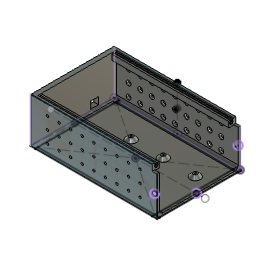
3U_Sliding_Nut (Autodesk Fusion 360 design; units mm, degrees)
Autodesk Fusion 360 part; units mm, degrees
note: some values were not read from the file. Set by a fixed rule: which face or edge a step refers to.
sketch "Sketch1" plane through (0, 0, 0) normal (0, 0, 1) x (1, 0, 0) in component "Case_Body"
  line L0 (96.52, 65) -> (-96.52, 65)
  line L1 (-96.52, 65) -> (-96.52, -65)
  line L2 (-96.52, -65) -> (96.52, -65)
  line L3 (96.52, -65) -> (96.52, 65)
  line L4 (96.52, 65) -> (-96.52, -65) construction
  line L5 (-96.52, 65) -> (96.52, -65) construction
  line L6 (-104.52, 69) -> (-96.52, 69)
  line L7 (-96.52, 69) -> (-96.52, -69)
  line L8 (-96.52, -69) -> (-104.52, -69)
  line L9 (-104.52, -69) -> (-104.52, 69)
  line L10 (-104.52, 69) -> (-96.52, -69) construction
  line L11 (-96.52, 69) -> (-104.52, -69) construction
  line L12 (-140, 0) -> (115, 0) construction
  line L13 (96.52, -69) -> (-96.52, -69)
  line L14 (-96.52, -69) -> (-96.52, -65)
  line L15 (-96.52, -65) -> (96.52, -65)
  line L16 (96.52, -65) -> (96.52, -69)
  line L17 (-96.52, 65) -> (96.52, 65)
  line L18 (-96.52, 69) -> (-96.52, 65)
  line L19 (96.52, 65) -> (96.52, 69)
  line L20 (-96.52, 65) -> (96.52, 65)
  line L21 (96.52, 69) -> (-96.52, 69)
  line L22 (104.52, 65) -> (96.52, 65)
  line L23 (96.52, 65) -> (96.52, -65)
  line L24 (96.52, -65) -> (104.52, -65)
  line L25 (104.52, -65) -> (104.52, 65)
  line L26 (104.52, 65) -> (96.52, -65) construction
  line L27 (96.52, 65) -> (104.52, -65) construction
  line L28 (104.52, 69) -> (96.52, 69)
  line L29 (96.52, 69) -> (96.52, 65)
  line L30 (96.52, 65) -> (104.52, 65)
  line L31 (104.52, 65) -> (104.52, 69)
  line L32 (96.52, -65) -> (104.52, -65)
  line L33 (104.52, -65) -> (104.52, -69)
  line L34 (104.52, -69) -> (96.52, -69)
  line L35 (96.52, -69) -> (96.52, -65)
  point P0 (-100.52, 0)
  point P1 (100.52, 0)
  dimension "d8" = 130
  dimension "d9" = 193.04
  dimension "d10" = 138
  dimension "d11" = 8
  dimension "d12" = 4
  dimension "d14" = 8
  dimension "d15" = 130
  constraint horizontal L0
  constraint perpendicular L0 L1
  constraint parallel L0 L2
  constraint parallel L1 L3
  constraint coincident L4 origin
  constraint coincident L5 origin
  constraint horizontal L6
  constraint perpendicular L6 L7
  constraint parallel L6 L8
  constraint parallel L7 L9
  constraint coincident L10 P0
  constraint coincident L11 P0
  constraint perpendicular L7 L12
  constraint coincident origin L12
  constraint coincident P0 L12
  constraint collinear L1 L7
  constraint horizontal L13
  constraint vertical L14
  constraint horizontal L15
  constraint vertical L16
  constraint coincident L1.end L2.start
  constraint symmetric L1.end L12 L0.end
  constraint symmetric L2.end L12 L0.start
  constraint symmetric L12 L13.start L19.end
  constraint symmetric L12 L7.end L6.end
  constraint symmetric L12 L1.end L0.end
  constraint symmetric L12 L2.end L0.start
  constraint horizontal L22
  constraint perpendicular L22 L23
  constraint parallel L22 L24
  constraint parallel L23 L25
  constraint coincident L26 P1
  constraint coincident L27 P1
  constraint coincident L12 P1
  constraint collinear L3 L23
  constraint horizontal L28
  constraint vertical L29
  constraint horizontal L30
  constraint vertical L31
  constraint coincident L0.start L3.end
  constraint coincident L22.start L25.end
  constraint coincident L19.end L21.start
  constraint horizontal L32
  constraint vertical L33
  constraint horizontal L34
  constraint vertical L35
  constraint coincident L2.end L3.start
  constraint coincident L13.start L16.end
  constraint coincident L24.end L25.start
  measures "d8" distance of L0.start L2.end
  measures "d9" distance of L0.start L0.end
  measures "d10" distance of L6.start L8.end
  measures "d11" distance of L7.end L8.end
  measures "d12" distance of L13.start L2.end
  measures "d14" distance of L22.start L0.start
  measures "d15" distance of L22.start L24.end
extrude "Extrude1" add sketch "Sketch1" along normal blind 4 contours L0 L1 L2 L3 L7 L15 L17 L20 L23 makes body 1 in component "Case_Body"
extrude "Extrude2" add sketch "Sketch1" along normal blind 74 contours L0 L7 L17 L18 L19 L20 L21 L29 | L1 L6 L7 L8 L9 L14 L18 | L2 L7 L13 L14 L15 L16 L35 bodies 1 in component "Case_Body"
extrude "Extrude3" add sketch "Sketch1" along normal blind 4 contours L3 L22 L23 L24 L25 L30 L32 bodies 1 in component "Case_Body"
extrude "Extrude4" add sketch "Sketch1" along normal blind 64 contours L19 L22 L28 L29 L30 L31 | L16 L24 L32 L33 L34 L35 bodies 1 in component "Case_Body"
ref_plane "WorkPlane1" through (104.52, 0, 32) normal (1, 0, 0) x (0, 1, 0) in component "Lid"
sketch "Sketch4" plane through (104.52, 0, 22) normal (1, 0, 0) x (0, 1, 0) in component "Lid"
  line L0 (-69, 42) -> (-65, 42)
  line L1 (-65, 42) -> (-65, 52)
  line L2 (-65, 52) -> (-69, 52)
  line L3 (-69, 52) -> (-69, 42)
  line L4 (65, 42) -> (69, 42)
  line L5 (69, 42) -> (69, 52)
  line L6 (69, 52) -> (65, 52)
  line L7 (65, 52) -> (65, 42)
  line L8 (-65, -18) -> (65, -18)
  line L9 (65, -18) -> (65, 52)
  line L10 (65, 52) -> (-65, 52)
  line L11 (-65, 52) -> (-65, -18)
extrude "Extrude1'" add sketch "Sketch4" against normal blind 8 separate body makes body 2 in component "Lid"
move_face "OffsetFaces1" offset -0.1 5 faces at (101.8533, -65, 44) (101.8533, -67.6667, 64) (99.1867, -21.6667, 4) (101.8533, 65, 24) (101.8533, 66.3333, 64) on bodies 2 in component "Lid"
sketch "Sketch5" plane through (0, 0, 4.1) normal (0, 0, -1) x (1, 0, 0) in component "Lid"
  line L0 (104.52, -64.9) -> (104.52, 64.9)
  line L1 (104.52, 64.9) -> (96.52, 64.9)
  line L2 (96.52, 64.9) -> (96.52, -64.9)
  line L3 (96.52, -64.9) -> (104.52, -64.9)
  line L4 (0, 0) -> (118, 0) construction
  circle A0 centre (100.52, 0) radius 1.25
  line L5 (100.52, 64.9) -> (100.52, -64.9) construction
  dimension "d29" = 2.5
  constraint coincident L4.start origin
  constraint perpendicular L2 L4
  constraint coincident L4 A0.centre
  constraint midpoint L1 L5.start
  constraint midpoint L3 L5.end
  constraint midpoint A0.centre L5
  measures "d29" diameter of A0
extrude "Extrude2'" cut sketch "Sketch5" against normal blind 10 contours A0 bodies 2 in component "Lid"
sketch "Sketch6" plane through (96.52, 0, 0) normal (-1, 0, 0) x (0, -1, 0) in component "Lid"
  line L0 (64.9, 64.1) -> (69, 64.1)
  line L1 (69, 64.1) -> (69, 74)
  line L2 (69, 74) -> (-69, 74)
  line L3 (-69, 74) -> (-69, 64.1)
  line L4 (-69, 64.1) -> (-64.9, 64.1)
  line L5 (-64.9, 64.1) -> (-64.9, 4.1)
  line L6 (-64.9, 4.1) -> (64.9, 4.1)
  line L7 (64.9, 4.1) -> (64.9, 64.1)
  line L8 (0, 0) -> (0, 41.8429) construction
  line L9 (2.55, 7.1) -> (-2.55, 7.1)
  line L10 (-2.55, 7.1) -> (-2.55, 5.5)
  line L11 (-2.55, 5.5) -> (2.55, 5.5)
  line L12 (2.55, 5.5) -> (2.55, 7.1)
  line L13 (2.55, 7.1) -> (-2.55, 5.5) construction
  line L14 (-2.55, 7.1) -> (2.55, 5.5) construction
  point P0 (0, 6.3)
  dimension "d33" = 1.6
  dimension "d34" = 3
  dimension "d35" = 5.1
  constraint coincident L8.start origin
  constraint perpendicular L6 L8
  constraint horizontal L9
  constraint perpendicular L9 L10
  constraint parallel L9 L11
  constraint parallel L10 L12
  constraint coincident L13 P0
  constraint coincident L14 P0
  constraint coincident L8 P0
  measures "d33" distance of L9.start L11.end
  measures "d34" distance of L6 L9
  measures "d35" distance of L9.start L9.end
extrude "Extrude3'" cut sketch "Sketch6" against normal blind 6.5 contours L9 L10 L11 L12 bodies 2 in component "Lid"
sketch "Sketch7" plane through (0, -64.9, 0) normal (0, -1, 0) x (1, 0, 0) in component "Lid"
  line L0 (104.52, 4.1) -> (104.52, 64.1)
  line L1 (104.52, 64.1) -> (96.52, 64.1)
  line L2 (96.52, 64.1) -> (96.52, 4.1)
  line L3 (96.52, 4.1) -> (104.52, 4.1)
  line L4 (96.52, 64.1) -> (104.52, 4.1) construction
  line L5 (104.52, 64.1) -> (96.52, 4.1) construction
  circle A0 centre (100.52, 34.1) radius 1.25
  dimension "d38" = 2.5
  constraint coincident L1.end L2.start
  constraint coincident L0.start L3.end
  constraint coincident L0.end L1.start
  constraint coincident L2.end L3.start
  constraint midpoint L4 A0.centre
  measures "d38" diameter of A0
extrude "Extrude4'" cut sketch "Sketch7" against normal blind 10 contours A0 bodies 2 in component "Lid"
sketch "Sketch8" plane through (96.52, 0, 0) normal (-1, 0, 0) x (0, -1, 0) in component "Lid"
  line L0 (-2.55, 7.1) -> (2.55, 7.1)
  line L1 (2.55, 7.1) -> (2.55, 5.5)
  line L2 (2.55, 5.5) -> (-2.55, 5.5)
  line L3 (-2.55, 5.5) -> (-2.55, 7.1)
  line L4 (64.9, 64.1) -> (69, 64.1)
  line L5 (69, 64.1) -> (69, 74)
  line L6 (69, 74) -> (-69, 74)
  line L7 (-69, 74) -> (-69, 64.1)
  line L8 (-69, 64.1) -> (-64.9, 64.1)
  line L9 (-64.9, 64.1) -> (-64.9, 4.1)
  line L10 (-64.9, 4.1) -> (64.9, 4.1)
  line L11 (64.9, 4.1) -> (64.9, 64.1)
  line L12 (64.9, 64.1) -> (64.9, 4.1) construction
  line L13 (61.9, 31.55) -> (63.5, 31.55)
  line L14 (63.5, 31.55) -> (63.5, 36.65)
  line L15 (63.5, 36.65) -> (61.9, 36.65)
  line L16 (61.9, 36.65) -> (61.9, 31.55)
  line L17 (61.9, 31.55) -> (63.5, 36.65) construction
  line L18 (63.5, 31.55) -> (61.9, 36.65) construction
  line L19 (89.3617, 34.1) -> (40.4383, 34.1) construction
  point P0 (62.7, 34.1)
  dimension "d42" = 1.6
  dimension "d43" = 5.1
  dimension "d81" = 3
  constraint coincident L4.start L11.end
  constraint coincident L10.end L11.start
  constraint horizontal L13
  constraint perpendicular L13 L14
  constraint parallel L13 L15
  constraint parallel L14 L16
  constraint coincident L17 P0
  constraint coincident L18 P0
  constraint perpendicular L11 L19
  constraint midpoint L12 L19
  constraint coincident P0 L19
  measures "d42" distance of L14.end L15.end
  measures "d43" distance of L13.end L14.end
  measures "d81" distance of L12 L15.end
extrude "Extrude5" cut sketch "Sketch8" against normal blind 6.5 contours L13 L14 L15 L16 bodies 2 in component "Lid"
mirror "Mirror1" about plane through (0, 0, 0) normal (0, 1, 0) of "Extrude4'", "Extrude5" in component "Lid"
sketch "Sketch2" plane through (0, 69, 0) normal (0, 1, 0) x (-1, 0, 0) in component "Case_Body"
  line L0 (-89.28, 0) -> (89.28, 0)
  line L1 (89.28, 0) -> (89.28, 54)
  line L2 (89.28, 54) -> (-81.28, 54)
  line L3 (-81.28, 54) -> (-81.28, 44)
  line L4 (-81.28, 44) -> (-89.28, 44)
  line L5 (-89.28, 44) -> (-89.28, 0)
  line L6 (-85.28, 44) -> (-85.28, -6) construction
  circle A0 centre (-85.28, 24.1) radius 1.25
  constraint midpoint L4 L6.start
  constraint perpendicular L0 L6
extrude "Extrude5'" [suppressed] in component "Case_Body"
chamfer "Chamfer1" [suppressed] in component "Case_Body"
mirror "Mirror1'" [suppressed] in component "Case_Body"
sketch "Sketch3" plane through (0, 0, 0) normal (0, 0, -1) x (1, 0, 0) in component "Case_Body"
  line L0 (89.28, -69) -> (89.28, 69)
  line L1 (89.28, 69) -> (-89.28, 69)
  line L2 (-89.28, 69) -> (-89.28, -69)
  line L3 (-89.28, -69) -> (89.28, -69)
  circle A0 centre (85.28, 0) radius 1.25
  point P0 (85.28, 0)
  dimension "d53" = 2.5
  constraint coincident P0 A0.centre
  measures "d53" diameter of A0
extrude "Extrude6" [suppressed] in component "Case_Body"
chamfer "Chamfer2" [suppressed] in component "Case_Body"
sketch "Sketch4 (2)" plane through (0, 0, 74) normal (0, 0, 1) x (-1, 0, 0) in component "Case_Body"
  line L0 (96.52, -65) -> (-96.52, -65)
  line L1 (-96.52, -65) -> (-96.52, -69)
  line L2 (-96.52, -69) -> (104.52, -69)
  line L3 (104.52, -69) -> (104.52, 69)
  line L4 (104.52, 69) -> (-96.52, 69)
  line L5 (-96.52, 69) -> (-96.52, 65)
  line L6 (-96.52, 65) -> (96.52, 65)
  line L7 (96.52, 65) -> (96.52, -65)
sketch "Sketch5 (2)" plane through (-96.52, 0, 0) normal (1, 0, 0) x (0, 1, 0) in component "Case_Body"
  line L0 (-65, 4) -> (65, 4)
  line L1 (65, 4) -> (65, 74)
  line L2 (65, 74) -> (-65, 74)
  line L3 (-65, 74) -> (-65, 4)
  line L4 (65, 72) -> (63.475, 72)
  line L5 (63.475, 72) -> (63.475, 69.97)
  line L6 (63.475, 69.97) -> (64.675, 69.97)
  line L7 (64.675, 69.97) -> (64.675, 67.87)
  line L8 (64.675, 67.87) -> (63.475, 67.87)
  line L9 (63.475, 67.87) -> (63.475, 66)
  line L10 (63.475, 66) -> (60.525, 66)
  line L11 (60.525, 66) -> (60.525, 67.87)
  line L12 (60.525, 67.87) -> (59.325, 67.87)
  line L13 (59.325, 67.87) -> (59.325, 69.97)
  line L14 (59.325, 69.97) -> (60.525, 69.97)
  line L15 (60.525, 69.97) -> (60.525, 72)
  line L16 (60.525, 72) -> (57.525, 72)
  line L17 (57.525, 72) -> (57.525, 63)
  line L18 (57.525, 63) -> (65, 63)
  line L19 (62, 66) -> (62, 78) construction
  point P0 (65, 74)
  dimension "d61" = 2
  dimension "d62" = 2.95
  dimension "d64" = 2.03
  dimension "d65" = 2.1
  dimension "d66" = 6
  dimension "d68" = 2.95
  dimension "d69" = 5.35
  dimension "d70" = 2.03
  dimension "d71" = 9
  dimension "d73" = 3
  dimension "d79" = 3
  constraint perpendicular L1 L4
  constraint perpendicular L4 L5
  constraint perpendicular L5 L6
  constraint perpendicular L4 L7
  constraint perpendicular L7 L8
  constraint perpendicular L8 L9
  constraint perpendicular L9 L10
  constraint perpendicular L10 L11
  constraint perpendicular L10 L13
  constraint perpendicular L13 L14
  constraint perpendicular L14 L15
  constraint perpendicular L15 L16
  constraint perpendicular L14 L17
  constraint coincident L1 L4.start
  constraint coincident L1 L18.end
  constraint collinear L4 L16
  constraint collinear L5 L9
  constraint horizontal L12
  constraint collinear L8 L12
  constraint midpoint L10 L19.start
  constraint perpendicular L2 L19
  constraint symmetric L7 L13 L19
  constraint horizontal L18
  measures "d61" distance of L4.start P0
  measures "d62" distance of L4.end L15.end
  measures "d64" distance of L4.end L5.end
  measures "d65" distance of L6.end L7.end
  measures "d66" distance of L4.end L9.end
  measures "d68" distance of L9.end L10.end
  measures "d69" distance of L7 L13
  measures "d70" distance of L14.end L15.end
  measures "d71" distance of L16.end L17.end
  measures "d73" distance of L15.end L16.end
  measures "d79" distance of L4.start L19
extrude "Extrude7" add sketch "Sketch5 (2)" along normal up to surface (193.04 mm away) contours L1 L4 L5 L6 L7 L8 L9 L10 L11 L12 L13 L14 L15 L16 L17 L18 bodies 1 in component "Case_Body"
mirror "Mirror2" about plane through (0, 0, 0) normal (0, 1, 0) of "Extrude7" in component "Case_Body"
chamfer "Chamfer3" distance 0.6 angle 45 1 faces at (-34.84, -23, 0) on bodies 1 in component "Case_Body"
sketch "Sketch6 (2)" plane through (0, 0, 0) normal (0, 0, -1) x (1, 0, 0) in component "Case_Body"
  line L0 (103.92, -68.4) -> (103.92, 68.4)
  line L1 (103.92, 68.4) -> (-103.92, 68.4)
  circle A0 centre (100.52, 0) radius 1.25
  line L2 (-103.92, 68.4) -> (-103.92, -68.4)
  line L3 (-103.92, -68.4) -> (103.92, -68.4)
extrude "Extrude8" cut sketch "Sketch6 (2)" against normal up to surface (4 mm away) contours A0 bodies 1 in component "Case_Body"
chamfer "Chamfer4" distance 2 angle 45 1 edges at (99.3546, -0.452, 0) on bodies 1 in component "Case_Body"
sketch "Sketch7 (2)" plane through (0, -69, 0) normal (0, -1, 0) x (1, 0, 0) in component "Case_Body"
  line L0 (-104.52, 0.6) -> (104.52, 0.6)
  line L1 (104.52, 0.6) -> (104.52, 64)
  line L2 (104.52, 64) -> (96.52, 64)
  line L3 (96.52, 64) -> (96.52, 74)
  line L4 (96.52, 74) -> (-104.52, 74)
  circle A0 centre (100.52, 34.1) radius 1.25
  line L5 (-104.52, 74) -> (-104.52, 0.6)
extrude "Extrude9" cut sketch "Sketch7 (2)" against normal up to surface (4 mm away) contours A0 bodies 1 in component "Case_Body"
chamfer "Chamfer5" distance 2 angle 45 1 edges at (99.3546, -69, 34.552) on bodies 1 in component "Case_Body"
mirror "Mirror3" about plane through (0, 0, 0) normal (0, 1, 0) of 2 faces at (103.0477, -68.5556, 32.8827) (100.1219, -65.6667, 35.2849) on bodies 1 in component "Case_Body"
chamfer "Chamfer6" distance 0.6 angle 45 4 edges at (104.52, -69, 32.3) (-104.52, -69, 37.3) (-104.52, 69, 37.3) (104.52, 69, 32.3) on bodies 1 in component "Case_Body"
chamfer "Chamfer7" distance 0.6 angle 45 3 edges at (-3.7, -69, 74) (-3.7, 69, 74) (-104.52, 0, 74) on bodies 1 in component "Case_Body"
fillet "Fillet1" radius 6 2 edges at (100.52, -64.9, 4.1) (100.52, 64.9, 4.1) on bodies 2 in component "Lid"
fillet "Fillet2" radius 6 2 edges at (4, -65, 4) (4, 65, 4) on bodies 1 in component "Case_Body"
chamfer "Chamfer1'" distance 0.6 angle 45 5 edges at (104.52, 69, 69.05) (100.52, 69, 74) (104.52, 0, 74) (104.52, -69, 69.05) (100.52, -69, 74) on bodies 2 in component "Lid"
sketch "Sketch8 (2)" plane through (0, 69, 0) normal (0, 1, 0) x (-1, 0, 0) in component "Case_Body"
  line L0 (103.92, 73.4) -> (-96.52, 73.4)
  line L1 (-96.52, 73.4) -> (-96.52, 64)
  line L2 (-96.52, 64) -> (-103.92, 64)
  line L3 (-103.92, 0.6) -> (103.92, 0.6)
  line L4 (0, 0) -> (0, 73.4) construction
  circle A0 centre (0, 36.7) radius 2
  line L5 (-103.92, 64) -> (-103.92, 0.6)
  line L6 (103.92, 0.6) -> (103.92, 73.4)
  circle A1 centre (-100.52, 34.1) radius 3.25
  dimension "d129" = 4
  constraint coincident L4.start origin
  constraint perpendicular L3 L4
  constraint coincident L4 A0.centre
  constraint midpoint L4 A0.centre
  constraint coincident L0 L4.end
  measures "d129" diameter of A0
extrude "Extrude10" cut sketch "Sketch8 (2)" against normal up to surface (4 mm away) contours A0 bodies 1 in component "Case_Body"
pattern_linear "R-Pattern1" count 9 spacing 19.13 along (1, 0, 0) both ways count 3 spacing 20 along (0, 0, -1) both ways of "Extrude10" in component "Case_Body"
mirror "Mirror4" about plane through (0, 0, 0) normal (0, 1, 0) of "Extrude10", "R-Pattern1" in component "Case_Body"
fillet "Fillet3" radius 2 54 edges at (1.8647, 65, 35.9768) (-74.6553, 65, 55.9768) (-74.6553, 65, 35.9768) (-74.6553, 65, 15.9768) (-55.5253, 65, 55.9768) (-55.5253, 65, 35.9768) (-55.5253, 65, 15.9768) (-36.3953, 65, 55.9768) (-36.3953, 65, 35.9768) (-36.3953, 65, 15.9768) (-17.2653, 65, 55.9768) (-17.2653, 65, 35.9768) (-17.2653, 65, 15.9768) (1.8647, 65, 55.9768) (1.8647, 65, 15.9768) (20.9947, 65, 55.9768) (20.9947, 65, 35.9768) (20.9947, 65, 15.9768) (40.1247, 65, 55.9768) (40.1247, 65, 35.9768) (40.1247, 65, 15.9768) (59.2547, 65, 55.9768) (59.2547, 65, 35.9768) (59.2547, 65, 15.9768) (78.3847, 65, 55.9768) (78.3847, 65, 35.9768) (78.3847, 65, 15.9768) (78.3847, -65, 55.9768) (78.3847, -65, 35.9768) (78.3847, -65, 15.9768) (59.2547, -65, 55.9768) (59.2547, -65, 35.9768) (59.2547, -65, 15.9768) (40.1247, -65, 55.9768) (40.1247, -65, 35.9768) (40.1247, -65, 15.9768) (20.9947, -65, 55.9768) (20.9947, -65, 35.9768) (20.9947, -65, 15.9768) (1.8647, -65, 15.9768) (1.8647, -65, 35.9768) (1.8647, -65, 55.9768) (-17.2653, -65, 55.9768) (-17.2653, -65, 35.9768) (-17.2653, -65, 15.9768) (-36.3953, -65, 55.9768) (-36.3953, -65, 35.9768) (-36.3953, -65, 15.9768) (-55.5253, -65, 55.9768) (-55.5253, -65, 35.9768) (-55.5253, -65, 15.9768) (-74.6553, -65, 55.9768) (-74.6553, -65, 35.9768) (-74.6553, -65, 15.9768) on bodies 1 in component "Case_Body"
sketch "Sketch3 (2)" plane through (0, 0, 4) normal (0, 0, 1) x (1, 0, 0) in component "Power PCB"
  line L0 (98.78, 39) -> (-96.22, 39)
  line L1 (-96.22, 39) -> (-96.22, 9)
  line L2 (-96.22, 9) -> (98.78, 9)
  line L3 (98.78, 9) -> (98.78, 39)
  line L4 (-104.22, 35) -> (-88.22, 35)
  line L5 (-88.22, 35) -> (-88.22, 23)
  line L6 (-88.22, 23) -> (-104.22, 23)
  line L7 (-104.22, 23) -> (-104.22, 35)
  circle A0 centre (-26.22, 19) radius 1.5
  circle A1 centre (26.78, 19) radius 1.5
  circle A2 centre (79.78, 19) radius 1.5
  line L8 (104.52, 59) -> (-96.52, 59)
  line L9 (-96.52, 59) -> (-96.52, -59)
  line L10 (-96.52, -59) -> (104.52, -59)
  line L11 (104.52, -59) -> (104.52, 59)
  circle A3 centre (100.52, 0) radius 1.25
  dimension "d145" = 195
  dimension "d146" = 30
  dimension "d147" = 16
  dimension "d148" = 12
  dimension "d149" = 8
  dimension "d150" = 4
  dimension "d156" = 70
  dimension "d157" = 10
  dimension "d158" = 3
  dimension "d159" = 3
  dimension "d160" = 3
  dimension "d161" = 53
  dimension "d162" = 10
  dimension "d163" = 53
  dimension "d164" = 10
  dimension "d167" = 0.3
  dimension "d188" = 20
  constraint horizontal L0
  constraint perpendicular L0 L1
  constraint parallel L0 L2
  constraint parallel L1 L3
  constraint horizontal L4
  constraint vertical L5
  constraint horizontal L6
  constraint vertical L7
  measures "d145" distance of L0.start L0.end
  measures "d146" distance of L0.start L2.end
  measures "d147" distance of L4.start L4.end
  measures "d148" distance of L4.start L6.end
  measures "d149" horizontal distance of L0.end L4.start
  measures "d150" vertical distance of L0.end L4.start
  measures "d156" distance of L1 A0.centre
  measures "d157" distance of L2 A0.centre
  measures "d158" diameter of A0
  measures "d159" diameter of A1
  measures "d160" diameter of A2
  measures "d161" horizontal distance of A0.centre A1.centre
  measures "d162" distance of L2 A1.centre
  measures "d163" distance of A1.centre A2.centre
  measures "d164" distance of L2 A2.centre
  measures "d167" distance of L1 L9
  measures "d188" distance of L0 L8
extrude "Extrude2''" add sketch "Sketch3 (2)" along normal blind 1.6 from surface at 5 separate body contours L0 L1 L2 L3 L4 L5 L6 | A0 | A1 | A2 makes body 3 in component "Power PCB"
extrude "Extrude3''" add sketch "Sketch3 (2)" along normal blind 10 from surface at 6.6 contours L1 L4 L5 L6 | L1 L4 L6 L9 | L4 L6 L7 L9 bodies 3 in component "Power PCB"
extrude "Extrude4''" cut sketch "Sketch3 (2)" along normal up to surface (6.6 mm away) contours A0 | A1 | A2 bodies 3 in component "Power PCB"
sketch "Sketch9" plane through (-96.52, 0, 0) normal (1, 0, 0) x (0, 1, 0) in component "Case_Body"
  arc A0 (59, 4) -> (65, 10) centre (59, 10) ccw
  line L0 (65, 10) -> (65, 63)
  line L1 (65, 63) -> (57.525, 63)
  line L2 (57.525, 63) -> (57.525, 72)
  line L3 (57.525, 72) -> (60.525, 72)
  line L4 (60.525, 72) -> (60.525, 69.97)
  line L5 (60.525, 69.97) -> (59.325, 69.97)
  line L6 (59.325, 69.97) -> (59.325, 67.87)
  line L7 (59.325, 67.87) -> (60.525, 67.87)
  line L8 (60.525, 67.87) -> (60.525, 66)
  line L9 (60.525, 66) -> (63.475, 66)
  line L10 (63.475, 66) -> (63.475, 67.87)
  line L11 (63.475, 67.87) -> (64.675, 67.87)
  line L12 (64.675, 67.87) -> (64.675, 69.97)
  line L13 (64.675, 69.97) -> (63.475, 69.97)
  line L14 (63.475, 69.97) -> (63.475, 72)
  line L15 (63.475, 72) -> (65, 72)
  line L16 (65, 72) -> (65, 74)
  line L17 (65, 74) -> (-65, 74)
  line L18 (-65, 74) -> (-65, 72)
  line L19 (-65, 72) -> (-63.475, 72)
  line L20 (-63.475, 72) -> (-63.475, 69.97)
  line L21 (-63.475, 69.97) -> (-64.675, 69.97)
  line L22 (-64.675, 69.97) -> (-64.675, 67.87)
  line L23 (-64.675, 67.87) -> (-63.475, 67.87)
  line L24 (-63.475, 67.87) -> (-63.475, 66)
  line L25 (-63.475, 66) -> (-60.525, 66)
  line L26 (-60.525, 66) -> (-60.525, 67.87)
  line L27 (-60.525, 67.87) -> (-59.325, 67.87)
  line L28 (-59.325, 67.87) -> (-59.325, 69.97)
  line L29 (-59.325, 69.97) -> (-60.525, 69.97)
  line L30 (-60.525, 69.97) -> (-60.525, 72)
  line L31 (-60.525, 72) -> (-57.525, 72)
  line L32 (-57.525, 72) -> (-57.525, 63)
  line L33 (-57.525, 63) -> (-65, 63)
  line L34 (-65, 63) -> (-65, 10)
  arc A1 (-65, 10) -> (-59, 4) centre (-59, 10) ccw
  line L35 (-59, 4) -> (59, 4)
  line L36 (35, 10.6) -> (35, 20.6)
  line L37 (35, 20.6) -> (23, 20.6)
  line L38 (23, 20.6) -> (23, 10.6)
  line L39 (23, 20.6) -> (35, 20.6)
  line L40 (35, 20.6) -> (35, 10.6)
  line L41 (35, 10.6) -> (23, 10.6)
  line L42 (23, 10.6) -> (23, 20.6)
  line L43 (23, 10.6) -> (35, 10.6)
  line L44 (22.6, 22.15) -> (35.4, 22.15)
  line L45 (35.4, 22.15) -> (35.4, 10.6)
  line L46 (35.4, 10.6) -> (22.6, 10.6)
  line L47 (22.6, 10.6) -> (22.6, 22.15)
  line L48 (23, 10.6) -> (35, 10.6)
  dimension "d209" = 1.55
  dimension "d210" = 0.4
  dimension "d211" = 0.4
  constraint horizontal L39
  constraint vertical L40
  constraint vertical L42
  constraint coincident L36.start L40.end
  constraint coincident L37.end L38.start
  constraint horizontal L44
  constraint vertical L45
  constraint horizontal L46
  constraint vertical L47
  constraint coincident L38.end L41.end
  constraint coincident L45.end L48
  measures "d209" distance of L39 L44
  measures "d210" distance of L42 L47
  measures "d211" distance of L40 L45
extrude "Extrude11" cut sketch "Sketch9" against normal up to surface (8 mm away) contours L36 L37 L38 L39 L40 L41 L42 L43 L46 L48 | L36 L37 L38 L39 L40 L42 L44 L45 L46 L47 bodies 1 in component "Case_Body"
sketch "Sketch10" plane through (0, 0, 4) normal (0, 0, 1) x (-1, 0, 0) in component "Case_Body"
  line L0 (-104.52, -59) -> (96.52, -59)
  line L1 (96.52, -59) -> (96.52, 59)
  line L2 (96.52, 59) -> (-104.52, 59)
  line L3 (-104.52, 59) -> (-104.52, -59)
  circle A0 centre (-100.52, 0) radius 1.25
  circle A1 centre (26.22, -19) radius 1.5
  circle A2 centre (-26.78, -19) radius 1.5
  circle A3 centre (-79.78, -19) radius 1.5
  circle A4 centre (26.22, -19) radius 3.5
  circle A5 centre (-26.78, -19) radius 3.5
  circle A6 centre (-79.78, -19) radius 3.5
  line L4 (96.52, -24) -> (-94.52, -24)
  line L5 (-94.52, -24) -> (-94.52, -14)
  line L6 (-94.52, -14) -> (96.52, -14)
  line L7 (96.52, -14) -> (96.52, -24)
  line L8 (-96.52, 65) -> (-96.52, -65)
  line L9 (-96.52, -65) -> (-96.52, 65)
  circle A7 centre (-26.78, -19) radius 1.25
  circle A8 centre (-79.78, -19) radius 1.25
  circle A9 centre (26.22, -19) radius 1.25
  dimension "d173" = 2
  dimension "d174" = 2
  dimension "d175" = 2
  dimension "d191" = 5
  dimension "d192" = 5
  dimension "d193" = 2
  dimension "d194" = -0.25
  dimension "d195" = -0.25
  dimension "d196" = -0.25
  constraint horizontal L4
  constraint vertical L5
  constraint horizontal L6
  constraint vertical L7
  constraint coincident L1 L4.start
  measures "d191" distance of A1.centre L4
  measures "d192" distance of A1.centre L6
  measures "d193" distance of L5 L9
extrude "Extrude12" add sketch "Sketch10" along normal up to surface (5 mm away) contours A1 | A2 | A3 | A4 | A5 | A6 bodies 1 in component "Case_Body"
sketch "Sketch9 (2)" plane through (96.52, 0, 0) normal (-1, 0, 0) x (0, -1, 0) in component "Lid"
  line L0 (-68.4, 74) -> (-69, 73.4)
  line L1 (-69, 73.4) -> (-69, 64.1)
  line L2 (-69, 64.1) -> (-64.9, 64.1)
  line L3 (-64.9, 64.1) -> (-64.9, 10.1)
  arc A0 (-64.9, 10.1) -> (-58.9, 4.1) centre (-58.9, 10.1) ccw
  line L4 (-58.9, 4.1) -> (58.9, 4.1)
  arc A1 (58.9, 4.1) -> (64.9, 10.1) centre (58.9, 10.1) ccw
  line L5 (64.9, 10.1) -> (64.9, 64.1)
  line L6 (64.9, 64.1) -> (69, 64.1)
  line L7 (69, 64.1) -> (69, 73.4)
  line L8 (69, 73.4) -> (68.4, 74)
  line L9 (68.4, 74) -> (-68.4, 74)
  line L10 (-2.55, 7.1) -> (2.55, 7.1)
  line L11 (2.55, 7.1) -> (2.55, 5.5)
  line L12 (2.55, 5.5) -> (-2.55, 5.5)
  line L13 (-2.55, 5.5) -> (-2.55, 7.1)
  line L14 (63.5, 31.55) -> (61.9, 31.55)
  line L15 (61.9, 31.55) -> (61.9, 36.65)
  line L16 (61.9, 36.65) -> (63.5, 36.65)
  line L17 (63.5, 36.65) -> (63.5, 31.55)
  line L18 (-61.9, 31.55) -> (-63.5, 31.55)
  line L19 (-63.5, 31.55) -> (-63.5, 36.65)
  line L20 (-63.5, 36.65) -> (-61.9, 36.65)
  line L21 (-61.9, 36.65) -> (-61.9, 31.55)
  line L22 (-9, 10.6) -> (-39, 10.6)
  line L23 (-9, 9) -> (-39, 9)
  line L24 (-9, 9) -> (-9, 10.6)
  line L25 (-9, 9) -> (-39, 9)
  line L26 (-39, 9) -> (-39, 10.6)
  line L27 (-39, 10.6) -> (-9, 10.6)
  line L28 (-9, 10.6) -> (-9, 9)
  line L29 (-39, 9) -> (-39, 10.6)
  line L30 (-41, 13.1) -> (-7, 13.1)
  line L31 (-7, 13.1) -> (-7, 6.5)
  line L32 (-7, 6.5) -> (-41, 6.5)
  line L33 (-41, 6.5) -> (-41, 13.1)
  dimension "d180" = 2
  dimension "d181" = 2.5
  dimension "d182" = 2.5
  dimension "d183" = 2
  constraint horizontal L30
  constraint vertical L31
  constraint horizontal L32
  constraint vertical L33
  measures "d180" distance of L28 L31
  measures "d181" distance of L22 L30
  measures "d182" distance of L23 L32
  measures "d183" distance of L29 L33
extrude "Extrude6'" cut sketch "Sketch9 (2)" against normal blind 2 contours L22 L23 L24 L25 L26 L27 L28 L29 | L30 L31 L32 L33 bodies 2 in component "Lid"
sketch "Sketch10 (2)" plane through (98.52, 0, 0) normal (-1, 0, 0) x (0, -1, 0) in component "Lid"
  line L0 (-41, 6.5) -> (-7, 6.5)
  line L1 (-7, 6.5) -> (-7, 13.1)
  line L2 (-7, 13.1) -> (-41, 13.1)
  line L3 (-41, 13.1) -> (-41, 6.5)
fillet "Fillet2'" radius 2 1 faces at (98.52, 29.6667, 10.9) on bodies 2 in component "Lid"
chamfer "Chamfer9" distance 5 distance2 5 3 edges at (-22.9569, 17.7343, 4) (30.0431, 17.7343, 4) (83.0431, 17.7343, 4) measured on face at (11.3337, -34.1374, 4) measured on face at (11.3337, -34.1374, 4) measured on face at (11.3337, -34.1374, 4) on bodies 1 in component "Case_Body"
sketch "Sketch11" plane through (0, 0, 4) normal (0, 0, 1) x (-1, 0, 0) in component "Case_Body"
  circle A0 centre (-26.78, -19) radius 8.5
  line L0 (-104.52, -59) -> (96.52, -59)
  line L1 (96.52, -59) -> (96.52, 59)
  line L2 (96.52, 59) -> (-104.52, 59)
  line L3 (-104.52, 59) -> (-104.52, -59)
  circle A1 centre (-100.52, 0) radius 1.25
  circle A2 centre (26.22, -19) radius 8.5
  circle A3 centre (-79.78, -19) radius 8.5
  circle A4 centre (90, -17) radius 1.5
  dimension "d203" = 3
  measures "d203" diameter of A4
extrude "Extrude13" [suppressed] in component "Case_Body"
chamfer "Chamfer10" [suppressed] in component "Case_Body"
component "Case_Body" placed x (1, 0, 0) y (0, 1, 0) z (0, 0, 1) at (0, 0, 0)
component "Lid" placed x (1, 0, 0) y (0, 1, 0) z (0, 0, 1) at (0, 0, 0)
component "Power PCB" placed x (1, 0, 0) y (0, 1, 0) z (0, 0, 1) at (0, 0, 0)
equation "case_width_hp = 38"
equation "_hp = 5.08 mm"
equation "side_width = 8 mm"
equation "top_bottom_width = 4 mm"
equation "case_depth = 70 mm"
equation "case_height = 130 mm"
equation "base_height = 4 mm"
equation "d8 = case_height"
equation "d9 = case_width_hp * _hp"
equation "d10 = case_height + ( 2 * top_bottom_width )"
equation "d11 = side_width"
equation "d12 = top_bottom_width"
equation "d13 = ( case_width_hp * _hp )"
equation "d14 = side_width"
equation "d15 = case_height"
equation "d16 = base_height"
equation "d18 = case_depth + base_height"
equation "d20 = base_height"
equation "mating_height = 10 mm"
equation "d23 = ( base_height + case_depth - mating_height )"
equation "d26 = -side_width"
equation "case_screw_hole_diameter = 2.5 mm"
equation "d29 = case_screw_hole_diameter"
equation "case_screw_hole_depth = 10 mm"
equation "d31 = -case_screw_hole_depth"
equation "d36 = -( ( side_width / 2 ) + 2.5 mm )"
equation "d38 = case_screw_hole_diameter"
equation "d39 = -case_screw_hole_depth"
equation "d44 = -( ( side_width / 2 ) + 2.5 mm )"
equation "d52 = case_screw_chamfer"
equation "d53 = case_screw_hole_diameter"
equation "d56 = case_screw_chamfer"
equation "rail_slot_nut_width = 5.35 mm"
equation "rail_slot_nut_height = 2.1 mm"
equation "rail_slot_hole_width = 2.95 mm"
equation "rail_slot_hole_depth = 6 mm"
equation "d62 = rail_slot_hole_width"
equation "rail_slot_nut_depth = 2.03 mm"
equation "d64 = rail_slot_nut_depth"
equation "d65 = rail_slot_nut_height"
equation "d66 = rail_slot_hole_depth"
equation "d68 = rail_slot_hole_width"
equation "d69 = rail_slot_nut_width"
equation "d70 = rail_slot_nut_depth"
equation "d71 = rail_slot_hole_depth + 3 mm"
equation "case_screw_chamfer = 2 mm"
equation "lid_tolerance = 0.1 mm"
equation "d83 = -lid_tolerance"
equation "d84 = bottom_chamfer"
equation "bottom_chamfer = 0.6 mm"
equation "edge_chamfer = 0.6 mm"
equation "d119 = edge_chamfer"
equation "d120 = edge_chamfer"
equation "lid_fillet = 6 mm"
equation "d124 = lid_fillet"
equation "d126 = lid_fillet"
equation "d127 = edge_chamfer"
equation "vent_hole_diameter = 4 mm"
equation "d129 = vent_hole_diameter"
equation "d134 = ( ( case_width_hp * _hp ) / 2 ) - 20 mm"
equation "d135 = ( case_depth / 2 ) - 15 mm"
equation "d139 = vent_interior_fillet"
equation "vent_interior_fillet = 2 mm"
